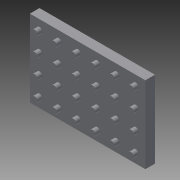
# Autodesk Inventor part: RectangularPattern
Saved by Autodesk Inventor 2015 (Build 190159000, 159)
## iProperties
Created: 2017-12-13
Part Number: RectangularPattern
Material: Generic
Document SubType Name: Modeling
Designer: Administrator
Density: 1 g/cm^3
Appearance: Default
Author: Administrator
Autodesk Inventor part; units mm, degrees
ref_plane "YZ Plane" through (0, 0, 0) normal (1, 0, 0) x (0, 1, 0)
ref_plane "XZ Plane" through (0, 0, 0) normal (0, 1, 0) x (-1, 0, 0)
ref_plane "XY Plane" through (0, 0, 0) normal (0, 0, 1) x (1, 0, 0)
sketch "Sketch1" plane through (0, 0, 0) normal (0, 0, 1) x (1, 0, 0)
  line L0 (1.5875, 101.6) -> (153.9875, 101.6)
  line L1 (153.9875, 101.6) -> (153.9875, 0)
  line L2 (153.9875, 0) -> (1.5875, 0)
  line L3 (1.5875, 0) -> (1.5875, 101.6)
  point P0 (0, 0)
  dimension "d0" = 101.6
  dimension "d1" = 152.4
  constraints: 8 end point, 2 parallel, 1 horizontal, 1 perpendicular
  measures "d0" distance of L2.end L0.start
  measures "d1" distance of L1.end L2.end
extrude "Extrusion1" add sketch "Sketch1" along normal blind 12.7
sketch "Sketch3" plane through (0, 0, 12.7) normal (0, 0, 1) x (1, 0, 0)
  circle A0 centre (14.2875, 12.7) radius 3.81
  line L0 (1.5875, 0) -> (1.5875, 101.6) projected
  line L1 (153.9875, 0) -> (1.5875, 0) projected
  circle A1 centre (14.2875, 38.1) radius 3.81
  circle A2 centre (14.2875, 63.5) radius 3.81
  circle A3 centre (14.2875, 88.9) radius 3.81
  circle A4 centre (39.6875, 12.7) radius 3.81
  circle A5 centre (39.6875, 38.1) radius 3.81
  circle A6 centre (39.6875, 63.5) radius 3.81
  circle A7 centre (39.6875, 88.9) radius 3.81
  circle A8 centre (65.0875, 12.7) radius 3.81
  circle A9 centre (65.0875, 38.1) radius 3.81
  circle A10 centre (65.0875, 63.5) radius 3.81
  circle A11 centre (65.0875, 88.9) radius 3.81
  circle A12 centre (90.4875, 12.7) radius 3.81
  circle A13 centre (90.4875, 38.1) radius 3.81
  circle A14 centre (90.4875, 63.5) radius 3.81
  circle A15 centre (90.4875, 88.9) radius 3.81
  circle A16 centre (115.8875, 12.7) radius 3.81
  circle A17 centre (115.8875, 38.1) radius 3.81
  circle A18 centre (115.8875, 63.5) radius 3.81
  circle A19 centre (115.8875, 88.9) radius 3.81
  circle A20 centre (141.2875, 12.7) radius 3.81
  circle A21 centre (141.2875, 38.1) radius 3.81
  circle A22 centre (141.2875, 63.5) radius 3.81
  circle A23 centre (141.2875, 88.9) radius 3.81
  point P0 (0, 0)
  dimension "d5" = 7.62
  dimension "d6" = 12.7
  dimension "d7" = 12.7
  dimension "d10" = 25.4
  dimension "d13" = 25.4
  constraints: 24 centre point, 1 horizontal, 1 vertical, 46 other
  measures "d5" diameter of A0
  measures "d6" distance from line of L0 A0.centre
  measures "d7" distance from line of L1 A0.centre
  measures "d10" distance of A0.centre A1.centre
  measures "d13" distance of A0.centre A4.centre
extrude "Extrusion2" add sketch "Sketch3" along normal blind 6.35
body "Solid1"
